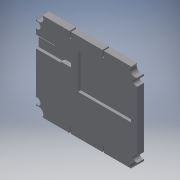
# Autodesk Inventor part: Каркас
Saved by Autodesk Inventor 2019 (Build 230136000, 136)
## iProperties
Created: 2020-05-20
Part Number: Каркас
Material: Типовые
Document SubType Name: Modeling
Designer: Surflay
Density: 1 g/cm^3
Appearance: По умолчанию
Author: Surflay
Autodesk Inventor part; units mm, degrees
ref_plane "YZ Plane" through (0, 0, 0) normal (1, 0, 0) x (0, 1, 0)
ref_plane "XZ Plane" through (0, 0, 0) normal (0, 1, 0) x (-1, 0, 0)
ref_plane "XY Plane" through (0, 0, 0) normal (0, 0, 1) x (1, 0, 0)
sketch "Эскиз1" plane through (0, 0, 0) normal (0, 0, 1) x (1, 0, 0)
  line L0 (174.3111, 41.624) -> (229.3111, 41.624) projected
  line L1 (229.3111, 41.624) -> (229.3111, 31.624) projected
  line L2 (229.3111, 31.624) -> (174.3111, 31.624) projected
  line L3 (174.3111, 41.624) -> (174.3111, 31.624) projected
  line L4 (149.3111, 46.624) -> (159.3111, 46.624) projected
  line L5 (149.3111, 46.624) -> (149.3111, 86.624) projected
  line L6 (149.3111, 86.624) -> (159.3111, 86.624) projected
  line L7 (159.3111, 86.624) -> (159.3111, 46.624) projected
  line L8 (134.3111, 31.624) -> (134.3111, 41.624) projected
  line L9 (134.3111, 31.624) -> (79.3111, 31.624) projected
  line L10 (79.3111, 31.624) -> (79.3111, 41.624) projected
  line L11 (79.3111, 41.624) -> (134.3111, 41.624) projected
  line L12 (231.3111, -8.7934) -> (231.3111, 82.0414) projected
  arc A0 (221.499, 103.624) -> (231.3111, 93.8118) centre (227.0611, 99.374) ccw projected
  line L13 (221.499, 103.624) -> (180.3111, 103.624) projected
  line L14 (180.3111, 103.624) -> (180.3111, 94.124) projected
  line L15 (180.3111, 94.124) -> (178.3111, 94.124) projected
  line L16 (178.3111, 94.124) -> (178.3111, 103.624) projected
  line L17 (178.3111, 103.624) -> (130.3111, 103.624) projected
  line L18 (130.3111, 103.624) -> (130.3111, 94.124) projected
  line L19 (130.3111, 94.124) -> (128.3111, 94.124) projected
  line L20 (128.3111, 94.124) -> (128.3111, 103.624) projected
  line L21 (128.3111, 103.624) -> (87.1233, 103.624) projected
  arc A1 (77.3111, 93.8118) -> (87.1233, 103.624) centre (81.5611, 99.374) ccw projected
  line L22 (77.3111, 91.2066) -> (77.3111, 93.8118) projected
  arc A2 (87.1233, -30.376) -> (77.3111, -20.5639) centre (81.5611, -26.126) ccw projected
  line L23 (128.3111, -30.376) -> (87.1233, -30.376) projected
  line L24 (128.3111, -30.376) -> (128.3111, -20.876) projected
  line L25 (128.3111, -20.876) -> (130.3111, -20.876) projected
  line L26 (130.3111, -20.876) -> (130.3111, -30.376) projected
  line L27 (178.3111, -30.376) -> (130.3111, -30.376) projected
  line L28 (178.3111, -30.376) -> (178.3111, -20.876) projected
  line L29 (178.3111, -20.876) -> (180.3111, -20.876) projected
  line L30 (180.3111, -20.876) -> (180.3111, -30.376) projected
  line L31 (221.499, -30.376) -> (180.3111, -30.376) projected
  arc A3 (231.3111, -20.5639) -> (221.499, -30.376) centre (227.0611, -26.126) ccw projected
  line L32 (159.3111, 26.624) -> (149.3111, 26.624) projected
  line L33 (159.3111, 26.624) -> (159.3111, -13.376) projected
  line L34 (159.3111, -13.376) -> (149.3111, -13.376) projected
  line L35 (149.3111, -13.376) -> (149.3111, 26.624) projected
  arc A4 (231.3111, 91.2066) -> (231.3111, 82.0414) centre (229.3111, 86.624) ccw projected
  arc A5 (77.3111, -17.9586) -> (77.3111, -8.7934) centre (79.3111, -13.376) ccw projected
  arc A6 (77.3111, 82.0414) -> (77.3111, 91.2066) centre (79.3111, 86.624) ccw projected
  arc A7 (231.3111, -8.7934) -> (231.3111, -17.9586) centre (229.3111, -13.376) ccw projected
  line L36 (231.3111, 91.2066) -> (231.3111, 93.8118) projected
  line L37 (77.3111, -8.7934) -> (77.3111, 82.0414) projected
  line L38 (77.3111, -20.5639) -> (77.3111, -17.9586) projected
  line L39 (231.3111, -20.5639) -> (231.3111, -17.9586) projected
  point P0 (0, 0)
  point P1 (251.3111, 35.624)
  point P2 (251.3111, 37.624)
  point P3 (57.3111, 37.624)
  point P4 (57.3111, 35.624)
  point P5 (179.3111, -20.876)
  point P6 (129.3111, -20.876)
  point P7 (70.835, 120.6534)
  point P8 (129.3111, 94.124)
  point P9 (179.3111, 94.124)
  point P10 (242.2845, 49.4059)
  point P11 (79.3111, -13.376)
  point P12 (229.3111, -13.376)
  constraints: 4 midpoint
extrude "Выдавливание1" add sketch "Эскиз1" along normal blind 10 contours L0 L1 L2 L3 | L5 L6 L7 L4 | L9 L10 L11 L8 | A7 L39 A3 L31 L30 L29 L28 L27 L26 L25 L24 L23 A2 L38 A5 L37 A6 L22 A1 L21 L20 L19 L18 L17 L16 L15 L14 L13 A0 L36 A4 L12 | L33 L34 L35 L32
sketch "Эскиз2" plane through (0, 0, 10) normal (0, 0, 1) x (1, 0, 0)
  line L0 (221.3111, 30.284) -> (141.3111, 30.284)
  line L1 (141.3111, 30.284) -> (141.3111, 83.624)
  line L2 (141.3111, 83.624) -> (221.3111, 83.624)
  line L3 (221.3111, 83.624) -> (221.3111, 30.284)
  line L4 (231.3111, -8.7934) -> (231.3111, 82.0414) projected
  line L5 (221.499, 103.624) -> (180.3111, 103.624) projected
  point P0 (0, 0)
  dimension "d14" = 80
  dimension "d15" = 53.34
  dimension "d58" = 20
  dimension "d59" = 10
  constraints: 8 end point, 2 parallel, 1 horizontal, 1 perpendicular
  measures "d14" distance of L0.start L0.end
  measures "d15" distance of L0.end L1.end
  measures "d58" distance between parallel lines of L5 L2
  measures "d59" distance between parallel lines of L4 L3
extrude "Выдавливание2" cut sketch "Эскиз2" against normal blind 4
